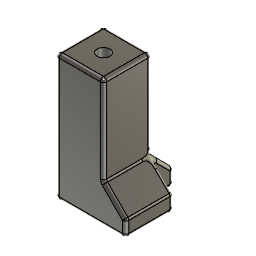
Foot_Front_Extended_Keyed (Autodesk Fusion 360 design; units mm, degrees)
Autodesk Fusion 360 part; units mm, degrees
sketch "Sketch1" plane through (0, 0, 0) normal (0, 0, 1) x (1, 0, 0)
  line L0 (7.5, 7.5) -> (-7.5, 7.5) construction
  line L1 (-7.5, 7.5) -> (-7.5, -7.5)
  line L2 (-7.5, -7.5) -> (7.5, -7.5)
  line L3 (7.5, -7.5) -> (7.5, 7.5) construction
  line L4 (7.5, 7.5) -> (-7.5, -7.5) construction
  line L5 (-7.5, 7.5) -> (7.5, -7.5) construction
  line L6 (7.5, 7.5) -> (14.5, 7.5)
  line L7 (14.5, 7.5) -> (14.5, -7.5)
  line L8 (14.5, -7.5) -> (7.5, -7.5)
  line L9 (7.5, -7.5) -> (7.5, 7.5) construction
  line L10 (-7.5, 7.5) -> (7.5, 7.5) construction
  line L11 (7.5, 7.5) -> (7.5, 14.5)
  line L12 (7.5, 14.5) -> (-7.5, 14.5)
  line L13 (-7.5, 14.5) -> (-7.5, 7.5)
  dimension "d1" = 15
  dimension "d4" = 22
  dimension "d5" = 15
  dimension "d6" = 22
  constraint horizontal L0
  constraint perpendicular L0 L1
  constraint parallel L0 L2
  constraint parallel L1 L3
  constraint coincident L4 origin
  constraint coincident L5 origin
  constraint horizontal L6
  constraint vertical L7
  constraint horizontal L8
  constraint vertical L9
  constraint horizontal L10
  constraint vertical L11
  constraint horizontal L12
  constraint vertical L13
  constraint equal L7 L12
  constraint equal L8 L13
  measures "d1" distance of L0.start L2.end
  measures "d4" distance of L1.end L12.end
  measures "d5" distance of L11.end L12.end
  measures "d6" distance of L1.end L7.end
extrude "Extrude1" add sketch "Sketch1" along normal blind 5
sketch "Sketch2" plane through (0, 0, 5) normal (0, 0, 1) x (-1, 0, 0)
  line L0 (-7.5, -7.5) -> (-7.5, -14.5)
  line L1 (-7.5, -14.5) -> (7.5, -14.5)
  line L2 (7.5, -14.5) -> (7.5, 7.5)
  line L3 (7.5, 7.5) -> (-14.5, 7.5)
  line L4 (-14.5, 7.5) -> (-14.5, -7.5)
  line L5 (-14.5, -7.5) -> (-7.5, -7.5)
  line L6 (-7.5, -7.5) -> (7.5, -7.5)
  line L7 (7.5, -7.5) -> (7.5, 7.5)
  line L8 (7.5, 7.5) -> (-7.5, 7.5)
  line L9 (-7.5, 7.5) -> (-7.5, -7.5)
  line L10 (-7.5, -7.5) -> (7.5, 7.5) construction
  line L11 (7.5, -7.5) -> (-7.5, 7.5) construction
  constraint horizontal L6
  constraint perpendicular L6 L7
  constraint parallel L6 L8
  constraint parallel L7 L9
  constraint coincident L0.start L5.end
  constraint coincident L10 origin
  constraint coincident L11 origin
extrude "Extrude2" add sketch "Sketch2" along normal blind 35 contours L2 L3 L6 L7 L8 L9
chamfer "Chamfer1" distance 7 angle 45 2 edges at (7.5, 0, 5) (0, 7.5, 5)
fillet "Fillet3" radius 1 12 faces at (-2.5, 4.8333, 0) (2.5, 14.5, 1.6667) (2.5, 7.5, 21.3333) (-2.5, 9.8333, 9.6667) (-7.5, -2.5, 17.3333) (-2.5, -7.5, 17.3333) (7.5, -2.5, 21.3333) (12.1667, -2.5, 7.3333) (14.5, 2.5, 1.6667) (9.8333, 7.5, 5.6667) (7.5, 9.8333, 5.6667) (2.5, -2.5, 40)
sketch "Sketch3" plane through (0, 0, 0) normal (0, 0, 1) x (1, 0, 0)
  circle A0 centre (0, 0) radius 2
  dimension "d12" = 4
  constraint coincident A0.centre origin
  measures "d12" diameter of A0
extrude "Extrude3" cut sketch "Sketch3" along normal through all
sketch "Sketch4" plane through (0, 0, 0) normal (0, 0, -1) x (1, 0, 0)
  circle A0 centre (0, 0) radius 2
  line L0 (1.45, -11) -> (-1.45, -11)
  line L1 (-1.45, -11) -> (-1.45, -3.5)
  line L2 (-1.45, -3.5) -> (1.45, -3.5)
  line L3 (1.45, -3.5) -> (1.45, -11)
  line L4 (1.45, -11) -> (-1.45, -3.5) construction
  line L5 (-1.45, -11) -> (1.45, -3.5) construction
  line L6 (0, 0) -> (0, -14.5) construction
  line L7 (3.5, -1.45) -> (3.5, 1.45)
  line L8 (0, 0) -> (14.5, 0) construction
  line L9 (11, 1.45) -> (3.5, -1.45) construction
  line L10 (3.5, 1.45) -> (11, 1.45)
  line L11 (11, -1.45) -> (3.5, -1.45)
  line L12 (11, -1.45) -> (3.5, 1.45) construction
  line L13 (11, 1.45) -> (11, -1.45)
  arc A1 (8.5, -6.5) -> (6.5, -8.5) centre (8.5, -8.5) ccw
  line L14 (8.5, -6.5) -> (13.5, -6.5)
  line L15 (13.5, -6.5) -> (13.5, 6.5)
  line L16 (13.5, 6.5) -> (-6.5, 6.5)
  line L17 (-6.5, 6.5) -> (-6.5, -13.5)
  line L18 (-6.5, -13.5) -> (6.5, -13.5)
  line L19 (6.5, -13.5) -> (6.5, -8.5)
  point P0 (0, -7.25)
  point P1 (7.25, 0)
  dimension "d14" = 2.9
  dimension "d15" = 7.5
  dimension "d17" = 90
  constraint horizontal L0
  constraint perpendicular L0 L1
  constraint parallel L0 L2
  constraint parallel L1 L3
  constraint coincident L4 P0
  constraint coincident L5 P0
  constraint coincident A0.centre L6.start
  constraint coincident P0 L6
  constraint midpoint P0 L6
  measures "d14" distance of L1.end L2.end
  measures "d15" distance of L0.start L2.end
extrude "Extrude4" add sketch "Sketch4" along normal blind 2 contours L0 L1 L2 L3 | L7 L10 L11 L13
fillet "Fillet1" radius 0.25 8 edges at (0, 11, -2) (-1.45, 7.25, -2) (1.45, 7.25, -2) (0, 3.5, -2) (7.25, 1.45, -2) (3.5, 0, -2) (7.25, -1.45, -2) (11, 0, -2)
fillet "Fillet1" radius 0.25 8 edges at (1.45, 11, -1) (-1.45, 11, -1) (-1.45, 3.5, -1) (1.45, 3.5, -1) (3.5, 1.45, -1) (11, 1.45, -1) (3.5, -1.45, -1) (11, -1.45, -1)
fillet "Fillet2" radius 0.25 16 edges at (-1.3768, 3.5732, 0) (0, 3.5, 0) (1.3768, 3.5732, 0) (1.45, 7.25, 0) (1.3768, 10.9268, 0) (0, 11, 0) (-1.3768, 10.9268, 0) (-1.45, 7.25, 0) (3.5732, 1.3768, 0) (3.5, 0, 0) (3.5732, -1.3768, 0) (7.25, -1.45, 0) (10.9268, -1.3768, 0) (11, 0, 0) (10.9268, 1.3768, 0) (7.25, 1.45, 0)
